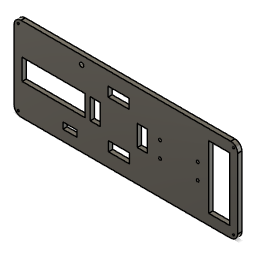
NEW_Top_Robot_Sanchez v28 (Autodesk Fusion 360 design; units mm, degrees)
Autodesk Fusion 360 part; units mm, degrees
sketch "Esquisse1" plane through (0, 0, 0) normal (0, 0, 1) x (1, 0, 0)
  circle A0 centre (-158.4581, 54) radius 1.41
  circle A1 centre (149.5419, -54) radius 1.41
  arc A2 (-164.4581, -50) -> (-154.4581, -60) centre (-154.4581, -50) ccw
  line L0 (-164.4581, -50) -> (-164.4581, 50)
  line L1 (145.5419, -60) -> (-154.4581, -60)
  circle A3 centre (149.5419, 54) radius 1.41
  arc A4 (-154.4581, 60) -> (-164.4581, 50) centre (-154.4581, 50) ccw
  line L2 (-154.4581, 60) -> (145.5419, 60)
  arc A5 (145.5419, -60) -> (155.5419, -50) centre (145.5419, -50) ccw
  arc A6 (155.5419, 50) -> (145.5419, 60) centre (145.5419, 50) ccw
  circle A7 centre (-158.4581, -54) radius 1.41
  line L3 (155.5419, -50) -> (155.5419, 50)
  line L4 (-62.9581, -14.994) -> (-62.9581, 15.006)
  line L5 (-152.9581, 15.006) -> (-62.9581, 15.006)
  line L6 (-152.9581, 15.006) -> (-152.9581, -14.994)
  line L7 (-152.9581, -14.994) -> (-62.9581, -14.994)
  line L8 (114.0419, 45.0068) -> (114.0419, -44.9932)
  line L9 (114.0419, -44.9932) -> (144.0419, -44.9932)
  line L10 (144.0419, -44.9932) -> (144.0419, 45.0068)
  line L11 (144.0419, 45.0068) -> (114.0419, 45.0068)
  line L12 (0, 0) -> (-1.1308, 0)
  circle A8 centre (98.3681, 10.929) radius 2
  circle A9 centre (44.3681, 10.929) radius 2
  circle A10 centre (44.3681, -12.071) radius 2
  circle A11 centre (98.3681, -12.071) radius 2
  line L13 (-94.4581, -36) -> (-74.4581, -36)
  line L14 (-74.4581, -36) -> (-74.4581, -45)
  line L15 (-74.4581, -45) -> (-94.4581, -45)
  line L16 (-94.4581, -45) -> (-94.4581, -36)
  circle A12 centre (-67.8367, 48.1939) radius 3
  line L17 (-30.0666, 40.6396) -> (0.0544, 40.6396)
  line L18 (0.0544, 26.9019) -> (-30.0666, 26.9019)
  line L19 (-30.0666, 26.9019) -> (-30.0666, 40.6396)
  line L20 (0.0544, 40.6396) -> (0.0544, 26.9019)
  line L21 (-55.5354, 14.7224) -> (-41.2741, 14.7224)
  line L22 (-41.2741, 14.7224) -> (-41.2741, -15.1543)
  line L23 (-41.2741, -15.1543) -> (-55.5354, -15.1543)
  line L24 (-55.5354, -15.1543) -> (-55.5354, 14.7224)
  line L25 (-29.4785, -26.7458) -> (0.6425, -26.7458)
  line L26 (0.6425, -26.7458) -> (0.6425, -40.4835)
  line L27 (0.6425, -40.4835) -> (-29.4785, -40.4835)
  line L28 (-29.4785, -40.4835) -> (-29.4785, -26.7458)
  line L29 (11.85, 15.3104) -> (26.1113, 15.3104)
  line L30 (26.1113, 15.3104) -> (26.1113, -14.5663)
  line L31 (26.1113, -14.5663) -> (11.85, -14.5663)
  line L32 (11.85, -14.5663) -> (11.85, 15.3104)
  point P0 (-104.4581, 0)
  dimension "d10" = 10
  dimension "d11" = 10
  dimension "d12" = 10
  dimension "d29" = 30
  dimension "d30" = 90
  dimension "d31" = 30
  dimension "d32" = 30
  dimension "d136" = 20
  dimension "d137" = 9
  dimension "d166" = 6
  constraint horizontal L1
  constraint perpendicular L0 L1
  constraint parallel L1 L2
  constraint tangent L1 A5
  constraint tangent A6 L3
  constraint perpendicular L5 L6
  constraint perpendicular L6 L7
  constraint perpendicular L8 L11
  constraint perpendicular L8 L9
  constraint perpendicular L4 L5
  constraint perpendicular L10 L11
  constraint coincident L12.start origin
  constraint horizontal L12
  constraint horizontal L13
  constraint vertical L14
  constraint horizontal L15
  constraint vertical L16
  constraint horizontal L17
  constraint horizontal L18
  constraint vertical L19
  constraint perpendicular L18 L20
  constraint horizontal L21
  constraint vertical L22
  constraint horizontal L23
  constraint vertical L24
  constraint horizontal L25
  constraint vertical L26
  constraint horizontal L27
  constraint vertical L28
  constraint horizontal L29
  constraint vertical L30
  constraint horizontal L31
  constraint vertical L32
  measures "d10" radius of A5
  measures "d11" radius of A2
  measures "d12" radius of A4
  measures "d29" distance of L5.start L6.end
  measures "d30" distance of L4.start L6.end
  measures "d31" distance of L10.end L8.start
  measures "d32" distance of L8.end L9.end
  measures "d136" distance of L13.start L13.end
  measures "d137" distance of L13.start L15.end
  measures "d166" diameter of A12
extrude "Extrusion1" add sketch "Esquisse1" along normal blind 6 contours A2 L0 L1 A4 L2 A5 A6 L3 | L4 L5 L6 L7 | L8 L9 L10 L11 | A8 | A9 | A10 | A11 | L13 L14 L15 L16 | A12 | L17 L18 L19 L20 | L21 L22 L23 L24 | L25 L26 L27 L28 | L29 L30 L31 L32
extrude "Extrusion2" cut sketch "Esquisse1" along normal blind 6 contours L4 L5 L6 L7 | L8 L9 L10 L11
extrude "Extrusion6" cut sketch "Esquisse1" along normal blind 6 contours A8 | A9 | A10 | A11
extrude "Extrusion27" cut sketch "Esquisse1" along normal up to surface (6 mm away) contours L13 L14 L15 L16
extrude "Extrusion28" cut sketch "Esquisse1" along normal up to surface (6 mm away) contours A12
extrude "Extrusion29" cut sketch "Esquisse1" along normal up to surface (6 mm away) contours L17 L18 L19 L20 | L21 L22 L23 L24 | L25 L26 L27 L28 | L29 L30 L31 L32
named bodies: "Part 1"
